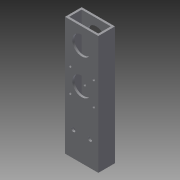
# Autodesk Inventor part: Z-ArmStructure
Saved by Autodesk Inventor 2013 (Build 170138000, 138)
## iProperties
Created: 2014-01-22
Part Number: Z-ArmStructure
Material: Generic
Document SubType Name: Modeling
Designer: Jarod
Density: 1 g/cm^3
Author: Jarod
Autodesk Inventor part; units mm, degrees
ref_plane "YZ Plane" through (0, 0, 0) normal (1, 0, 0) x (0, 1, 0)
ref_plane "XZ Plane" through (0, 0, 0) normal (0, 1, 0) x (-1, 0, 0)
ref_plane "XY Plane" through (0, 0, 0) normal (0, 0, 1) x (1, 0, 0)
sketch "Sketch1" plane through (0, 0, 0) normal (0, 1, 0) x (-1, 0, 0)
  line L0 (25.4, 12.7) -> (-25.4, 12.7)
  line L1 (-25.4, 12.7) -> (-25.4, -12.7)
  line L2 (-25.4, -12.7) -> (25.4, -12.7)
  line L3 (25.4, -12.7) -> (25.4, 12.7)
  line L4 (25.4, 12.7) -> (-25.4, -12.7) construction
  line L5 (-25.4, 12.7) -> (25.4, -12.7) construction
  line L6 (22.225, 9.525) -> (-22.225, 9.525)
  line L7 (-22.225, 9.525) -> (-22.225, -9.525)
  line L8 (-22.225, -9.525) -> (22.225, -9.525)
  line L9 (22.225, -9.525) -> (22.225, 9.525)
  line L10 (22.225, 9.525) -> (-22.225, -9.525) construction
  line L11 (-22.225, 9.525) -> (22.225, -9.525) construction
  point P0 (0, 0)
  dimension "d0" = 50.8
  dimension "d1" = 25.4
  dimension "d2" = 44.45
  dimension "d3" = 19.05
  constraints: 24 end point, 4 midpoint, 4 parallel, 2 horizontal, 2 perpendicular
  measures "d0" distance of L2.end L1.end
  measures "d1" distance of L1.end L0.end
  measures "d2" distance of L8.end L7.end
  measures "d3" distance of L7.end L6.end
extrude "Extrusion1" add sketch "Sketch1" along normal blind 180.975
sketch "Sketch2" plane through (25.4, 0, -12.7) normal (0, 0, -1) x (-1, 0, 0)
  line L0 (50.8, 0) -> (50.8, 180.975) projected
  line L1 (0, 180.975) -> (50.8, 180.975) projected
  line L2 (0, 0) -> (0, 180.975) projected
  line L3 (25.4, 0) -> (63.5, 0) construction
  line L4 (25.4, 38.1) -> (50.8, 38.1)
  line L5 (50.8, 38.1) -> (0, 38.1)
  line L6 (0, 38.1) -> (12.7, 38.1)
  line L7 (0, 38.1) -> (12.7, 38.1) construction
  line L8 (12.7, 38.1) -> (38.1, 38.1)
  circle A0 centre (12.7, 38.1) radius 3.175
  circle A1 centre (38.1, 38.1) radius 3.175
  line L9 (25.4, 180.975) -> (25.4, 155.575)
  line L10 (25.4, 180.975) -> (50.8, 180.975) construction
  circle A2 centre (25.4, 155.575) radius 14.2875
  dimension "d6" = 38.1
  dimension "d8" = 12.7
  dimension "d9" = 0
  dimension "d10" = 25.4
  dimension "d11" = 180
  dimension "d12" = 6.35
  dimension "d13" = 6.35
  dimension "d14" = 25.4
  dimension "d15" = 90
  dimension "d16" = 28.575
  constraints: 16 end point, 3 centre point, 3 coincident, 3 horizontal, 2 collinear, 2 equal length, 2 perpendicular, 2 point on line, 1 midpoint
  measures "d6" distance of L3.start L4.start
  measures "d8" distance of L5.end L6.end
  measures "d9" distance between parallel lines of L6 L7
  measures "d10" distance of L6.end L8.end
  measures "d11" angle of L8 L6
  measures "d12" diameter of A0
  measures "d13" diameter of A1
  measures "d14" distance of L9.start L9.end
  measures "d15" angle of L9 L10
  measures "d16" diameter of A2
extrude "Extrusion2" cut sketch "Sketch2" against normal blind 180.975 contours A2 | A1 L4 | L4 A1 | A0 L5 | L5 A0
sketch "Sketch3" plane through (25.4, 0, -12.7) normal (0, 0, -1) x (-1, 0, 0)
  line L0 (0, 0) -> (0, 180.975) projected
  line L1 (25.4, 0) -> (25.4, 101.6)
  line L2 (25.4, 0) -> (127, 0) construction
  circle A0 centre (25.4, 101.6) radius 14.2875
  line L3 (25.4, 101.6) -> (43.3605, 119.5605)
  line L4 (25.4, 101.6) -> (50.8, 101.6) construction
  line L5 (43.3605, 119.5605) -> (7.4395, 83.6395)
  line L6 (7.4395, 83.6395) -> (43.3605, 83.6395)
  line L7 (43.3605, 83.6395) -> (43.3605, 119.5605)
  line L8 (43.3605, 119.5605) -> (7.4395, 119.5605)
  line L9 (7.4395, 119.5605) -> (7.4395, 83.6395)
  circle A1 centre (7.4395, 119.5605) radius 2.032
  circle A2 centre (43.3605, 119.5605) radius 2.032
  circle A3 centre (43.3605, 83.6395) radius 2.032
  circle A4 centre (7.4395, 83.6395) radius 2.032
  dimension "d19" = 101.6
  dimension "d20" = 90
  dimension "d21" = 28.575
  dimension "d22" = 25.4
  dimension "d23" = 45
  dimension "d24" = 50.8
  dimension "d25" = 0
  dimension "d26" = 4.064
  dimension "d27" = 4.064
  dimension "d28" = 4.064
  dimension "d29" = 4.064
  constraints: 18 end point, 5 centre point, 5 coincident, 3 horizontal, 3 parallel, 2 equal length, 1 collinear, 1 perpendicular
  measures "d19" distance of L1.start L1.end
  measures "d20" angle of L2 L1
  measures "d21" diameter of A0
  measures "d22" distance of L3.start L3.end
  measures "d23" angle of L4 L3
  measures "d24" distance of L3.end L5.end
  measures "d25" distance between parallel lines of L5 L3
  measures "d26" diameter of A1
  measures "d27" diameter of A2
  measures "d28" diameter of A3
  measures "d29" diameter of A4
extrude "Extrusion3" cut sketch "Sketch3" against normal blind 180.975 contours A0 L5 L1 | L1 L3 A0 | A4 L9 L6 | L6 L5 A4 | A3 L7 L6 | L6 L7 A3 | L5 A0 L3 | L9 A4 L5 | A1 L8 L9 | L9 L8 A1 | A2 L3 L7 | L7 L8 A2 | A2 L8 L3
body "Solid1"
